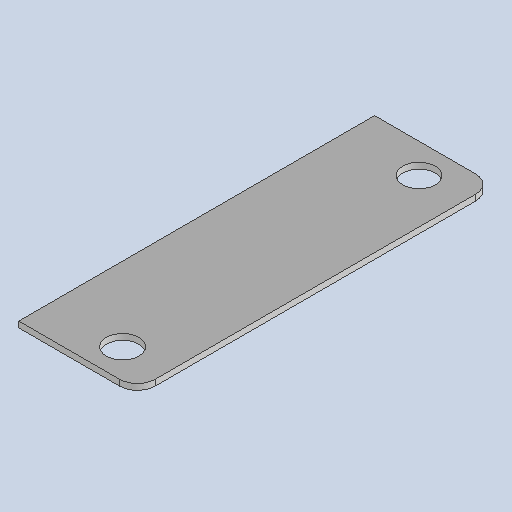
# Autodesk Inventor part: TRM 023 face damper
Saved by Autodesk Inventor 2025 (Build 290162010, 162A)
## iProperties
Created: 2024-08-07
Part Number: TRM 023 face damper
Material: AISI 304
Document SubType Name: Sheet Metal
Designer: pokla
Density: 8.02768 g/cm^3
Flat Pattern Width: 12 cm
Flat Pattern Length: 4 cm
Flat Pattern Area: 48 cm^2
Sheet Metal Rule: AISI304 2mm Die16
Sheet Metal Width: 120.000 mm
Sheet Metal Length: 40.000 mm
Sheet Metal Area: 4800.000 mm^2
Appearance: Default
Stock Number: ТРМ 023 лицо успокоитель
Mass: 73.7661 g
Surface Area: 99.5689 cm^2
Volume: 9.18896 cm^3
Author: pokla
Autodesk Inventor part; units mm, degrees
ref_plane "YZ Plane" through (0, 0, 0) normal (1, 0, 0) x (0, 1, 0)
ref_plane "XZ Plane" through (0, 0, 0) normal (0, 1, 0) x (-1, 0, 0)
ref_plane "XY Plane" through (0, 0, 0) normal (0, 0, 1) x (1, 0, 0)
sketch "Sketch1" plane through (0, 0, 0) normal (0, 0, 1) x (1, 0, 0)
  line L0 (-20, -60) -> (20, -60)
  line L1 (20, -60) -> (20, 60)
  line L2 (20, 60) -> (-20, 60)
  line L3 (-20, 60) -> (-20, -60)
  line L4 (-20, -60) -> (20, 60) construction
  line L5 (20, -60) -> (-20, 60) construction
  circle A0 centre (5, 50) radius 5.5
  circle A1 centre (5, -50) radius 5.5
  line L6 (-20, 0) -> (20, 0) construction
  point P0 (0, 0)
  point P1 (0, 0)
  dimension "d0" = 40
  dimension "d1" = 120
  dimension "d12" = 11
  dimension "d13" = 100
  dimension "d15" = 15
  measures "d0" distance of L2.end L1.end
  measures "d1" distance of L1.end L0.end
  measures "d12" diameter of A0
  measures "d13" distance of A1.centre A0.centre
  measures "d15" distance from line of A0.centre L1
extrude "Plate1" add sketch "Sketch1" along normal blind 2
sketch "Sketch2" plane through (0, 0, 0) normal (0, 0, -1) x (-1, 0, 0)
  line L0 (0, 40) -> (200, 40) construction
  line L1 (200, 40) -> (200, 20) construction
  line L2 (200, 20) -> (0, 20) construction
  line L3 (0, 20) -> (0, 40) construction
  line L4 (-20, 60) -> (20, 60) projected
  line L5 (-20, -60) -> (-20, 60) projected
  point P0 (0, 0)
  point P1 (-48, 100)
  point P2 (20, 60)
  point P3 (-50, 98)
  dimension "d6" = 200
  dimension "d9" = 20
  dimension "d10" = 20
  dimension "d11" = 20
  constraints: 4 other
  measures "d6" distance of L0.start L0.end
  measures "d9" distance of L0.end L1.end
  measures "d11" length of L3
mark "Mark1"
fillet "Corner Round1" radius 6 2 edges at (20, -60, 1) (20, 60, 1)
equation "\"d2\" = Thickness"
equation "\"BendReliefWidth\" = Thickness"
equation "\"BendReliefDepth\" = 0.5 * Thickness"
equation "\"CornerReliefSize\" = 4 * Thickness"
equation "\"MinimumRemnant\" = 2 * Thickness"
equation "\"TransitionRadius\" = BendRadius"
equation "\"JacobiRadiusSize\" = BendRadius"
equation "\"GapSize\" = Thickness"
equation "\"Thickness\" = 2"
equation "\"BendRadius\" = 2.75"
body "Solid1"
